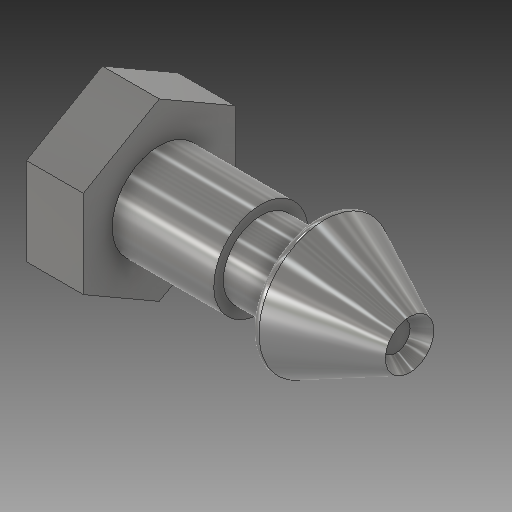
# Autodesk Inventor part: 212-05
Saved by Autodesk Inventor 2019 (Build 230136000, 136)
## iProperties
Company: Autodesk Inc.
Created: 2017-03-14
Part Number: 212-05
Material: Titanium
Document SubType Name: Modeling
Designer: Autodesk Inc.
Density: 4.51 g/cm^3
Appearance: Aluminum - Anodized Glossy (Grey)
Mass: 14.5425 g
Surface Area: 16.5776 cm^2
Volume: 3.22451 cm^3
Author: Inventor
Autodesk Inventor part; units mm, degrees
ref_plane "YZ Plane" through (0, 0, 0) normal (1, 0, 0) x (0, 1, 0)
ref_plane "XZ Plane" through (0, 0, 0) normal (0, 1, 0) x (-1, 0, 0)
ref_plane "XY Plane" through (0, 0, 0) normal (0, 0, 1) x (1, 0, 0)
sketch "Sketch1" plane through (0, 0, 0) normal (0, 0, 1) x (1, 0, 0)
  line L0 (0, 0) -> (26.387, 0)
  line L1 (0, 0) -> (0, 4.969)
  line L2 (0, 4.969) -> (10.717, 4.969)
  line L3 (10.717, 4.969) -> (10.717, 3.968)
  line L4 (10.717, 3.968) -> (16.717, 3.968)
  line L5 (16.717, 3.968) -> (16.717, 7.2744)
  line L6 (16.717, 7.2744) -> (26.387, 2.558)
  line L7 (26.387, 2.558) -> (24.9308, 1.5)
  line L8 (24.9308, 1.5) -> (24.9308, 0)
  dimension "d0" = 10.717
  dimension "d1" = 9.938
  dimension "d2" = 7.936
  dimension "d3" = 6
  dimension "d4" = 5.116
  dimension "d6" = 26
  dimension "d8" = 9.67
  dimension "d9" = 36
  dimension "d10" = 3
  constraints: 18 end point, 5 perpendicular, 1 horizontal, 1 point on line, 1 vertical
  measures "d0" distance of L1.end L2.end
  measures "d1" diameter of L2 L0
  measures "d2" diameter of L4 L0
  measures "d3" distance between parallel lines of L3 L5
  measures "d4" diameter of L6.end L0
  measures "d6" angle of L0 L6
  measures "d8" distance from line of L5 L6.end
  measures "d9" angle of L0 L7
  measures "d10" diameter of L7.end L0
revolve "Revolution1" add sketch "Sketch1" angle 360 about axis through (0, 0, 0) along (1, 0, 0)
sketch "Sketch2" plane through (0, 0, 0) normal (-1, 0, 0) x (0, 0, 1)
  circle A0 centre (0, 0) radius 4.969 projected
  line L0 (0, 9.2376) -> (8, 4.6188)
  line L1 (8, 4.6188) -> (8, -4.6188)
  line L2 (8, -4.6188) -> (0, -9.2376)
  line L3 (0, -9.2376) -> (-8, -4.6188)
  line L4 (-8, -4.6188) -> (-8, 4.6188)
  line L5 (-8, 4.6188) -> (0, 9.2376)
  dimension "d11" = 16
  constraints: 12 end point, 1 coincident, 1 vertical alignment, 13 other
  measures "d11" distance between parallel lines of L1 L4
extrude "Extrusion1" add sketch "Sketch2" along normal blind 6 contours A0 | L0 L1 L2 L3 L4 L5
fillet "Fillet1" radius 0.5 2 edges at (16.717, -3.968, 0) (16.717, -7.2744, 0)
body "Solid1"
